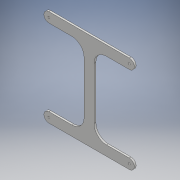
# Autodesk Inventor part: Handle 2
Saved by Autodesk Inventor 2018 (Build 220112000, 112)
## iProperties
Created: 2018-09-06
Part Number: Handle 2
Material: Generic
Document SubType Name: Modeling
Designer: matth
Density: 1 g/cm^3
Appearance: Default
Author: matth
Autodesk Inventor part; units mm, degrees
note: some values were not read from the file. Chosen so that the rebuilt part matches the saved one: sketch regions of "Extrusion1".
ref_plane "YZ Plane" through (0, 0, 0) normal (1, 0, 0) x (0, 1, 0)
ref_plane "XZ Plane" through (0, 0, 0) normal (0, 1, 0) x (-1, 0, 0)
ref_plane "XY Plane" through (0, 0, 0) normal (0, 0, 1) x (1, 0, 0)
sketch "Sketch1" plane through (0, 0, 0) normal (0, 1, 0) x (-1, 0, 0)
  line L0 (0, 0) -> (130, 0)
  line L1 (130, 0) -> (130, -140)
  line L2 (130, -140) -> (0, -140)
  line L3 (0, -140) -> (0, 0)
  circle A0 centre (0, 0) radius 1.5
  circle A1 centre (130, 0) radius 1.5
  circle A2 centre (130, -140) radius 1.5
  circle A3 centre (0, -140) radius 1.5
  circle A4 centre (0, -140) radius 8
  circle A5 centre (130, -140) radius 8
  circle A6 centre (130, 0) radius 8
  circle A7 centre (0, 0) radius 8
  line L4 (130, 0) -> (0, 0) construction
  line L5 (130, -8) -> (0, -8)
  line L6 (0, 8) -> (130, 8)
  arc A8 (130, -8) -> (130, 8) centre (130, 0) ccw
  arc A9 (0, 8) -> (0, -8) centre (0, 0) ccw
  line L7 (130, -140) -> (0, -140) construction
  line L8 (130, -148) -> (0, -148)
  line L9 (0, -132) -> (130, -132)
  arc A10 (130, -148) -> (130, -132) centre (130, -140) ccw
  arc A11 (0, -132) -> (0, -148) centre (0, -140) ccw
  line L10 (65, 0) -> (65, -70)
  line L11 (65, -140) -> (65, 0) construction
  line L12 (73, -140) -> (73, 0)
  line L13 (57, 0) -> (57, -140)
  arc A12 (57, -140) -> (73, -140) centre (65, -140) ccw
  arc A13 (73, 0) -> (57, 0) centre (65, 0) ccw
  dimension "d0" = 130
  dimension "d1" = 140
  dimension "d2" = 3
  dimension "d3" = 3
  dimension "d4" = 3
  dimension "d5" = 3
  dimension "d6" = 16
  dimension "d7" = 16
  dimension "d8" = 16
  dimension "d9" = 16
  dimension "d10" = 70
  dimension "d14" = 8
  constraints: 34 end point, 14 centre point, 12 point on circle, 12 tangent, 8 coincident, 7 equal length, 5 midpoint, 2 vertical, 1 concentric, 1 horizontal, 1 perpendicular
  measures "d0" distance of L1.end L2.end
  measures "d1" distance of L0.end L1.end
  measures "d2" diameter of A0
  measures "d3" diameter of A1
  measures "d4" diameter of A2
  measures "d5" diameter of A3
  measures "d6" diameter of A4
  measures "d7" diameter of A5
  measures "d8" diameter of A6
  measures "d9" diameter of A7
  measures "d10" distance of L10.start L10.end
  measures "d14" radius of A13
extrude "Extrusion1" add sketch "Sketch1" along normal blind 3 contours A0 L3 A7 L0 | L0 A7 L3 A0 | A7 L6 A13 L0 | L0 L13 L5 A7 | A13 L0 | L0 L10 L5 L13 | A4 L2 A3 L3 | L9 L13 L2 A4 | L3 A3 L2 A4 | L5 L12 L9 L13 | L0 L12 L5 L10 | L6 A6 L0 A13 | L2 A12 L8 A4 | L9 L12 L2 L13 | L0 A6 L5 L12 | A6 L1 A1 L0 | L2 A12 | A12 L2 A5 L8 | L9 A5 L2 L12 | L0 A1 L1 A6 | A5 L2 A2 L1 | L1 A2 L2 A5
fillet "Fillet1" radius 20 4 edges at (-57, 1.5, -132) (-73, 1.5, -132) (-57, 1.5, -8) (-73, 1.5, -8)
body "Solid1"
